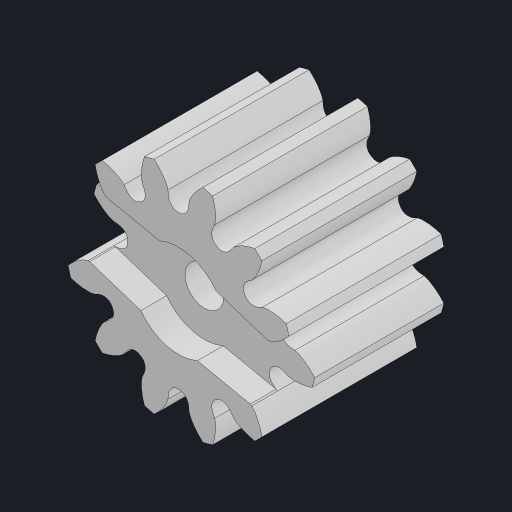
# Autodesk Inventor part: Servo Gear
Saved by Autodesk Inventor 2023.2 (Build 272271030, 271C)
## iProperties
Created: 2023-10-24
Part Number: Servo Gear
Material: Generic
Document SubType Name: Modeling
Designer: robpl
Density: 1 g/cm^3
Appearance: Default
Author: robpl
## iProperties of the stored document Servo Gear_3DPrint.ipt
Created: 2023-10-25
Part Number: Servo Gear_3DPrint
Material: Generic
Document SubType Name: Modeling
Designer: robpl
Density: 1 g/cm^3
Appearance: Default
Author: robpl
Autodesk Inventor part; units mm, degrees
ref_plane "YZ Plane" through (0, 0, 0) normal (1, 0, 0) x (0, 1, 0)
ref_plane "XZ Plane" through (0, 0, 0) normal (0, 1, 0) x (-1, 0, 0)
ref_plane "XY Plane" through (0, 0, 0) normal (0, 0, 1) x (1, 0, 0)
sketch "Sketch1" plane through (0, 0, 0) normal (0, 0, 1) x (1, 0, 0)
  spline S0 degree 3 poles (-1.8876, 8.544) (-1.8289, 8.4914) (-1.7116, 8.3861) (-1.5456, 8.2175) (-1.3882, 8.0411) (-1.2413, 7.8557) (-1.1064, 7.6613) (-1.0062, 7.4915) (-0.9353, 7.3507) (-0.8879, 7.2423) (-0.846, 7.1316) (-0.8276, 7.055) (-0.8183, 7.0166) knots 0 0 0 0 0.125009 0.250019 0.375027 0.500032 0.625031 0.75002 0.812526 0.87503 0.937528 1 1 1 1
  spline S1 degree 3 poles (-0.8183, 7.0166) (-0.8175, 6.9523) (-0.8164, 6.8558) (-0.8022, 6.7278) (-0.7847, 6.6329) (-0.763, 6.5388) (-0.732, 6.4474) (-0.6955, 6.358) (-0.6492, 6.2731) (-0.5944, 6.1935) (-0.5302, 6.1213) (-0.457, 6.058) (-0.3752, 6.0064) (-0.2866, 5.9676) (-0.1929, 5.943) (-0.0964, 5.9357) (0, 5.9384) (0.0964, 5.9357) (0.1929, 5.943) (0.2866, 5.9676) (0.3752, 6.0064) (0.457, 6.058) (0.5302, 6.1213) (0.5944, 6.1935) (0.6492, 6.2731) (0.6955, 6.358) (0.732, 6.4474) (0.763, 6.5388) (0.7847, 6.6329) (0.8022, 6.7278) (0.8164, 6.8558) (0.8175, 6.9523) (0.8183, 7.0166) knots 0 0 0 0 0.062509 0.093773 0.125034 0.156299 0.187559 0.218819 0.250082 0.281336 0.312585 0.343826 0.375061 0.406291 0.43751 0.468735 0.5 0.531265 0.56249 0.593709 0.624939 0.656174 0.687415 0.718664 0.749918 0.781181 0.812441 0.843701 0.874966 0.906227 0.937491 1 1 1 1
  spline S2 degree 3 poles (0.8183, 7.0166) (0.8276, 7.055) (0.846, 7.1316) (0.8879, 7.2423) (0.9353, 7.3507) (1.0062, 7.4915) (1.1064, 7.6613) (1.2413, 7.8557) (1.3882, 8.0411) (1.5456, 8.2175) (1.7116, 8.3861) (1.8289, 8.4914) (1.8876, 8.544) knots 0 0 0 0 0.062472 0.12497 0.187474 0.24998 0.374969 0.499968 0.624973 0.749981 0.874991 1 1 1 1
  circle A0 centre (0, 0) radius 5.9375 construction
  circle A1 centre (0, 0) radius 7.0477 construction
  circle A2 centre (0, 0) radius 7.5 construction
  circle A3 centre (0, 0) radius 8.75
  point P0 (-1.7133, 8.3843)
  point P1 (-1.5471, 8.2162)
  point P2 (-1.3899, 8.0396)
  point P3 (-1.2433, 7.8542)
  point P4 (-1.1089, 7.6597)
  point P5 (-0.9893, 7.4559)
  point P6 (-0.9363, 7.3502)
  point P7 (-0.8889, 7.2419)
  point P8 (-0.8484, 7.1309)
  point P9 (-0.8118, 6.8239)
  point P10 (-0.8011, 6.728)
  point P11 (-0.784, 6.6331)
  point P12 (-0.7615, 6.5393)
  point P13 (-0.7311, 6.4477)
  point P14 (-0.6939, 6.3587)
  point P15 (-0.6478, 6.274)
  point P16 (-0.5928, 6.1948)
  point P17 (-0.5287, 6.1228)
  point P18 (-0.4555, 6.06)
  point P19 (-0.374, 6.0085)
  point P20 (-0.2857, 5.97)
  point P21 (-0.1924, 5.9459)
  point P22 (-0.0965, 5.9373)
  point P23 (0, 5.9375)
  point P24 (0.0965, 5.9373)
  point P25 (0.1924, 5.9459)
  point P26 (0.2857, 5.97)
  point P27 (0.374, 6.0085)
  point P28 (0.4555, 6.06)
  point P29 (0.5287, 6.1228)
  point P30 (0.5928, 6.1948)
  point P31 (0.6478, 6.274)
  point P32 (0.6939, 6.3587)
  point P33 (0.7311, 6.4477)
  point P34 (0.7615, 6.5393)
  point P35 (0.784, 6.6331)
  point P36 (0.8011, 6.728)
  point P37 (0.8118, 6.8239)
  point P38 (0.8484, 7.1309)
  point P39 (0.8889, 7.2419)
  point P40 (0.9363, 7.3502)
  point P41 (0.9893, 7.4559)
  point P42 (1.1089, 7.6597)
  point P43 (1.2433, 7.8542)
  point P44 (1.3899, 8.0396)
  point P45 (1.5471, 8.2162)
  point P46 (1.7133, 8.3843)
  constraints: 4 centre point, 2 point on circle, 109 other
extrude "Extrusion1" add sketch "Sketch1" against normal blind 10
extrude "Extrusion2" cut sketch "Sketch1" against normal through all contours A3 S2 S1 S0 picked at (-0.2347, 7.8651)
pattern_circular "Circular Pattern1" count 12 over 360 about axis through (0, 0, 0) along (0, 0, -1) of "Extrusion2"
sketch "Sketch3" plane through (0, 0, 0) normal (0, 0, 1) x (1, 0, 0)
  spline S0 degree 3 poles (-2.6372, 8.3431) (-2.6618, 8.2682) (-2.7108, 8.1184) (-2.7702, 7.8894) (-2.8183, 7.6579) (-2.8529, 7.4239) (-2.8725, 7.1881) (-2.8743, 6.9909) (-2.8653, 6.8335) (-2.8522, 6.716) (-2.8331, 6.5992) (-2.8108, 6.5235) (-2.7996, 6.4857) knots 0 0 0 0 0.125009 0.250019 0.375027 0.500032 0.625031 0.75002 0.812526 0.87503 0.937528 1 1 1 1 projected
  spline S1 degree 3 poles (-2.7996, 6.4857) (-2.7681, 6.4296) (-2.7209, 6.3455) (-2.6692, 6.2276) (-2.6369, 6.1366) (-2.6086, 6.0443) (-2.5897, 5.9496) (-2.5766, 5.8539) (-2.5743, 5.7573) (-2.582, 5.661) (-2.6015, 5.5663) (-2.6333, 5.4749) (-2.6783, 5.3893) (-2.7356, 5.3114) (-2.8045, 5.2433) (-2.8843, 5.1886) (-2.9692, 5.1428) (-3.0513, 5.0922) (-3.1386, 5.0504) (-3.232, 5.0248) (-3.3281, 5.0141) (-3.4248, 5.0179) (-3.5198, 5.0361) (-3.6115, 5.0666) (-3.6988, 5.1081) (-3.7813, 5.1584) (-3.8576, 5.2176) (-3.9302, 5.2813) (-3.996, 5.3519) (-4.0586, 5.4254) (-4.1349, 5.5291) (-4.1842, 5.6121) (-4.217, 5.6674) knots 0 0 0 0 0.062509 0.093773 0.125034 0.156299 0.187559 0.218819 0.250082 0.281336 0.312585 0.343826 0.375061 0.406291 0.43751 0.468735 0.5 0.531265 0.56249 0.593709 0.624939 0.656174 0.687415 0.718664 0.749918 0.781181 0.812441 0.843701 0.874966 0.906227 0.937491 1 1 1 1 projected
  spline S2 degree 3 poles (-4.217, 5.6674) (-4.2442, 5.696) (-4.2985, 5.7531) (-4.3902, 5.8281) (-4.4853, 5.8982) (-4.6172, 5.9847) (-4.7889, 6.0817) (-5.0028, 6.1826) (-5.2227, 6.2697) (-5.4473, 6.3438) (-5.6753, 6.4068) (-5.8296, 6.4393) (-5.9067, 6.4555) knots 0 0 0 0 0.062472 0.12497 0.187474 0.24998 0.374969 0.499968 0.624973 0.749981 0.874991 1 1 1 1 projected
  arc A0 (-5.9067, 6.4555) -> (-6.4555, 5.9067) centre (0, 0) ccw projected
  spline S3 degree 3 poles (-6.4555, 5.9067) (-6.4393, 5.8296) (-6.4068, 5.6753) (-6.3438, 5.4473) (-6.2697, 5.2227) (-6.1826, 5.0028) (-6.0817, 4.7889) (-5.9847, 4.6172) (-5.8982, 4.4853) (-5.8281, 4.3902) (-5.7531, 4.2985) (-5.696, 4.2442) (-5.6674, 4.217) knots 0 0 0 0 0.125009 0.250019 0.375027 0.500032 0.625031 0.75002 0.812526 0.87503 0.937528 1 1 1 1 projected
  spline S4 degree 3 poles (-5.6674, 4.217) (-5.6121, 4.1842) (-5.5291, 4.1349) (-5.4254, 4.0586) (-5.3519, 3.996) (-5.2813, 3.9302) (-5.2176, 3.8576) (-5.1584, 3.7813) (-5.1081, 3.6988) (-5.0666, 3.6115) (-5.0361, 3.5198) (-5.0179, 3.4248) (-5.0141, 3.3281) (-5.0248, 3.232) (-5.0504, 3.1386) (-5.0922, 3.0513) (-5.1428, 2.9692) (-5.1886, 2.8843) (-5.2433, 2.8045) (-5.3114, 2.7356) (-5.3893, 2.6783) (-5.4749, 2.6333) (-5.5663, 2.6015) (-5.661, 2.582) (-5.7573, 2.5743) (-5.8539, 2.5766) (-5.9496, 2.5897) (-6.0443, 2.6086) (-6.1366, 2.6369) (-6.2276, 2.6692) (-6.3455, 2.7209) (-6.4296, 2.7681) (-6.4857, 2.7996) knots 0 0 0 0 0.062509 0.093773 0.125034 0.156299 0.187559 0.218819 0.250082 0.281336 0.312585 0.343826 0.375061 0.406291 0.43751 0.468735 0.5 0.531265 0.56249 0.593709 0.624939 0.656174 0.687415 0.718664 0.749918 0.781181 0.812441 0.843701 0.874966 0.906227 0.937491 1 1 1 1 projected
  arc A1 (-8.3431, 2.6372) -> (-8.544, 1.8876) centre (0, 0) ccw projected
  spline S5 degree 3 poles (-7.0166, 0.8183) (-6.9523, 0.8175) (-6.8558, 0.8164) (-6.7278, 0.8022) (-6.6329, 0.7847) (-6.5388, 0.763) (-6.4474, 0.732) (-6.358, 0.6955) (-6.2731, 0.6492) (-6.1935, 0.5944) (-6.1213, 0.5302) (-6.058, 0.457) (-6.0064, 0.3752) (-5.9676, 0.2866) (-5.943, 0.1929) (-5.9357, 0.0964) (-5.9384, 0) (-5.9357, -0.0964) (-5.943, -0.1929) (-5.9676, -0.2866) (-6.0064, -0.3752) (-6.058, -0.457) (-6.1213, -0.5302) (-6.1935, -0.5944) (-6.2731, -0.6492) (-6.358, -0.6955) (-6.4474, -0.732) (-6.5388, -0.763) (-6.6329, -0.7847) (-6.7278, -0.8022) (-6.8558, -0.8164) (-6.9523, -0.8175) (-7.0166, -0.8183) knots 0 0 0 0 0.062509 0.093773 0.125034 0.156299 0.187559 0.218819 0.250082 0.281336 0.312585 0.343826 0.375061 0.406291 0.43751 0.468735 0.5 0.531265 0.56249 0.593709 0.624939 0.656174 0.687415 0.718664 0.749918 0.781181 0.812441 0.843701 0.874966 0.906227 0.937491 1 1 1 1 projected
  spline S6 degree 3 poles (-7.0166, -0.8183) (-7.055, -0.8276) (-7.1316, -0.846) (-7.2423, -0.8879) (-7.3507, -0.9353) (-7.4915, -1.0062) (-7.6613, -1.1064) (-7.8557, -1.2413) (-8.0411, -1.3882) (-8.2175, -1.5456) (-8.3861, -1.7116) (-8.4914, -1.8289) (-8.544, -1.8876) knots 0 0 0 0 0.062472 0.12497 0.187474 0.24998 0.374969 0.499968 0.624973 0.749981 0.874991 1 1 1 1 projected
  arc A2 (-8.544, -1.8876) -> (-8.3431, -2.6372) centre (0, 0) ccw projected
  spline S7 degree 3 poles (-8.3431, -2.6372) (-8.2682, -2.6618) (-8.1184, -2.7108) (-7.8894, -2.7702) (-7.6579, -2.8183) (-7.4239, -2.8529) (-7.1881, -2.8725) (-6.9909, -2.8743) (-6.8335, -2.8653) (-6.716, -2.8522) (-6.5992, -2.8331) (-6.5235, -2.8108) (-6.4857, -2.7996) knots 0 0 0 0 0.125009 0.250019 0.375027 0.500032 0.625031 0.75002 0.812526 0.87503 0.937528 1 1 1 1 projected
  spline S8 degree 3 poles (-6.4857, -2.7996) (-6.4296, -2.7681) (-6.3455, -2.7209) (-6.2276, -2.6692) (-6.1366, -2.6369) (-6.0443, -2.6086) (-5.9496, -2.5897) (-5.8539, -2.5766) (-5.7573, -2.5743) (-5.661, -2.582) (-5.5663, -2.6015) (-5.4749, -2.6333) (-5.3893, -2.6783) (-5.3114, -2.7356) (-5.2433, -2.8045) (-5.1886, -2.8843) (-5.1428, -2.9692) (-5.0922, -3.0513) (-5.0504, -3.1386) (-5.0248, -3.232) (-5.0141, -3.3281) (-5.0179, -3.4248) (-5.0361, -3.5198) (-5.0666, -3.6115) (-5.1081, -3.6988) (-5.1584, -3.7813) (-5.2176, -3.8576) (-5.2813, -3.9302) (-5.3519, -3.996) (-5.4254, -4.0586) (-5.5291, -4.1349) (-5.6121, -4.1842) (-5.6674, -4.217) knots 0 0 0 0 0.062509 0.093773 0.125034 0.156299 0.187559 0.218819 0.250082 0.281336 0.312585 0.343826 0.375061 0.406291 0.43751 0.468735 0.5 0.531265 0.56249 0.593709 0.624939 0.656174 0.687415 0.718664 0.749918 0.781181 0.812441 0.843701 0.874966 0.906227 0.937491 1 1 1 1 projected
  spline S9 degree 3 poles (-5.6674, -4.217) (-5.696, -4.2442) (-5.7531, -4.2985) (-5.8281, -4.3902) (-5.8982, -4.4853) (-5.9847, -4.6172) (-6.0817, -4.7889) (-6.1826, -5.0028) (-6.2697, -5.2227) (-6.3438, -5.4473) (-6.4068, -5.6753) (-6.4393, -5.8296) (-6.4555, -5.9067) knots 0 0 0 0 0.062472 0.12497 0.187474 0.24998 0.374969 0.499968 0.624973 0.749981 0.874991 1 1 1 1 projected
  arc A3 (-6.4555, -5.9067) -> (-5.9067, -6.4555) centre (0, 0) ccw projected
  spline S10 degree 3 poles (-5.9067, -6.4555) (-5.8296, -6.4393) (-5.6753, -6.4068) (-5.4473, -6.3438) (-5.2227, -6.2697) (-5.0028, -6.1826) (-4.7889, -6.0817) (-4.6172, -5.9847) (-4.4853, -5.8982) (-4.3902, -5.8281) (-4.2985, -5.7531) (-4.2442, -5.696) (-4.217, -5.6674) knots 0 0 0 0 0.125009 0.250019 0.375027 0.500032 0.625031 0.75002 0.812526 0.87503 0.937528 1 1 1 1 projected
  spline S11 degree 3 poles (-4.217, -5.6674) (-4.1842, -5.6121) (-4.1349, -5.5291) (-4.0586, -5.4254) (-3.996, -5.3519) (-3.9302, -5.2813) (-3.8576, -5.2176) (-3.7813, -5.1584) (-3.6988, -5.1081) (-3.6115, -5.0666) (-3.5198, -5.0361) (-3.4248, -5.0179) (-3.3281, -5.0141) (-3.232, -5.0248) (-3.1386, -5.0504) (-3.0513, -5.0922) (-2.9692, -5.1428) (-2.8843, -5.1886) (-2.8045, -5.2433) (-2.7356, -5.3114) (-2.6783, -5.3893) (-2.6333, -5.4749) (-2.6015, -5.5663) (-2.582, -5.661) (-2.5743, -5.7573) (-2.5766, -5.8539) (-2.5897, -5.9496) (-2.6086, -6.0443) (-2.6369, -6.1366) (-2.6692, -6.2276) (-2.7209, -6.3455) (-2.7681, -6.4296) (-2.7996, -6.4857) knots 0 0 0 0 0.062509 0.093773 0.125034 0.156299 0.187559 0.218819 0.250082 0.281336 0.312585 0.343826 0.375061 0.406291 0.43751 0.468735 0.5 0.531265 0.56249 0.593709 0.624939 0.656174 0.687415 0.718664 0.749918 0.781181 0.812441 0.843701 0.874966 0.906227 0.937491 1 1 1 1 projected
  spline S12 degree 3 poles (-2.7996, -6.4857) (-2.8108, -6.5235) (-2.8331, -6.5992) (-2.8522, -6.716) (-2.8653, -6.8335) (-2.8743, -6.9909) (-2.8725, -7.1881) (-2.8529, -7.4239) (-2.8183, -7.6579) (-2.7702, -7.8894) (-2.7108, -8.1184) (-2.6618, -8.2682) (-2.6372, -8.3431) knots 0 0 0 0 0.062472 0.12497 0.187474 0.24998 0.374969 0.499968 0.624973 0.749981 0.874991 1 1 1 1 projected
  arc A4 (-2.6372, -8.3431) -> (-1.8876, -8.544) centre (0, 0) ccw projected
  spline S13 degree 3 poles (-1.8876, -8.544) (-1.8289, -8.4914) (-1.7116, -8.3861) (-1.5456, -8.2175) (-1.3882, -8.0411) (-1.2413, -7.8557) (-1.1064, -7.6613) (-1.0062, -7.4915) (-0.9353, -7.3507) (-0.8879, -7.2423) (-0.846, -7.1316) (-0.8276, -7.055) (-0.8183, -7.0166) knots 0 0 0 0 0.125009 0.250019 0.375027 0.500032 0.625031 0.75002 0.812526 0.87503 0.937528 1 1 1 1 projected
  spline S14 degree 3 poles (-0.8183, -7.0166) (-0.8175, -6.9523) (-0.8164, -6.8558) (-0.8022, -6.7278) (-0.7847, -6.6329) (-0.763, -6.5388) (-0.732, -6.4474) (-0.6955, -6.358) (-0.6492, -6.2731) (-0.5944, -6.1935) (-0.5302, -6.1213) (-0.457, -6.058) (-0.3752, -6.0064) (-0.2866, -5.9676) (-0.1929, -5.943) (-0.0964, -5.9357) (0, -5.9384) (0.0964, -5.9357) (0.1929, -5.943) (0.2866, -5.9676) (0.3752, -6.0064) (0.457, -6.058) (0.5302, -6.1213) (0.5944, -6.1935) (0.6492, -6.2731) (0.6955, -6.358) (0.732, -6.4474) (0.763, -6.5388) (0.7847, -6.6329) (0.8022, -6.7278) (0.8164, -6.8558) (0.8175, -6.9523) (0.8183, -7.0166) knots 0 0 0 0 0.062509 0.093773 0.125034 0.156299 0.187559 0.218819 0.250082 0.281336 0.312585 0.343826 0.375061 0.406291 0.43751 0.468735 0.5 0.531265 0.56249 0.593709 0.624939 0.656174 0.687415 0.718664 0.749918 0.781181 0.812441 0.843701 0.874966 0.906227 0.937491 1 1 1 1 projected
  spline S15 degree 3 poles (0.8183, -7.0166) (0.8276, -7.055) (0.846, -7.1316) (0.8879, -7.2423) (0.9353, -7.3507) (1.0062, -7.4915) (1.1064, -7.6613) (1.2413, -7.8557) (1.3882, -8.0411) (1.5456, -8.2175) (1.7116, -8.3861) (1.8289, -8.4914) (1.8876, -8.544) knots 0 0 0 0 0.062472 0.12497 0.187474 0.24998 0.374969 0.499968 0.624973 0.749981 0.874991 1 1 1 1 projected
  arc A5 (1.8876, -8.544) -> (2.6372, -8.3431) centre (0, 0) ccw projected
  spline S16 degree 3 poles (2.6372, -8.3431) (2.6618, -8.2682) (2.7108, -8.1184) (2.7702, -7.8894) (2.8183, -7.6579) (2.8529, -7.4239) (2.8725, -7.1881) (2.8743, -6.9909) (2.8653, -6.8335) (2.8522, -6.716) (2.8331, -6.5992) (2.8108, -6.5235) (2.7996, -6.4857) knots 0 0 0 0 0.125009 0.250019 0.375027 0.500032 0.625031 0.75002 0.812526 0.87503 0.937528 1 1 1 1 projected
  spline S17 degree 3 poles (2.7996, -6.4857) (2.7681, -6.4296) (2.7209, -6.3455) (2.6692, -6.2276) (2.6369, -6.1366) (2.6086, -6.0443) (2.5897, -5.9496) (2.5766, -5.8539) (2.5743, -5.7573) (2.582, -5.661) (2.6015, -5.5663) (2.6333, -5.4749) (2.6783, -5.3893) (2.7356, -5.3114) (2.8045, -5.2433) (2.8843, -5.1886) (2.9692, -5.1428) (3.0513, -5.0922) (3.1386, -5.0504) (3.232, -5.0248) (3.3281, -5.0141) (3.4248, -5.0179) (3.5198, -5.0361) (3.6115, -5.0666) (3.6988, -5.1081) (3.7813, -5.1584) (3.8576, -5.2176) (3.9302, -5.2813) (3.996, -5.3519) (4.0586, -5.4254) (4.1349, -5.5291) (4.1842, -5.6121) (4.217, -5.6674) knots 0 0 0 0 0.062509 0.093773 0.125034 0.156299 0.187559 0.218819 0.250082 0.281336 0.312585 0.343826 0.375061 0.406291 0.43751 0.468735 0.5 0.531265 0.56249 0.593709 0.624939 0.656174 0.687415 0.718664 0.749918 0.781181 0.812441 0.843701 0.874966 0.906227 0.937491 1 1 1 1 projected
  spline S18 degree 3 poles (4.217, -5.6674) (4.2442, -5.696) (4.2985, -5.7531) (4.3902, -5.8281) (4.4853, -5.8982) (4.6172, -5.9847) (4.7889, -6.0817) (5.0028, -6.1826) (5.2227, -6.2697) (5.4473, -6.3438) (5.6753, -6.4068) (5.8296, -6.4393) (5.9067, -6.4555) knots 0 0 0 0 0.062472 0.12497 0.187474 0.24998 0.374969 0.499968 0.624973 0.749981 0.874991 1 1 1 1 projected
  arc A6 (5.9067, -6.4555) -> (6.4555, -5.9067) centre (0, 0) ccw projected
  spline S19 degree 3 poles (6.4555, -5.9067) (6.4393, -5.8296) (6.4068, -5.6753) (6.3438, -5.4473) (6.2697, -5.2227) (6.1826, -5.0028) (6.0817, -4.7889) (5.9847, -4.6172) (5.8982, -4.4853) (5.8281, -4.3902) (5.7531, -4.2985) (5.696, -4.2442) (5.6674, -4.217) knots 0 0 0 0 0.125009 0.250019 0.375027 0.500032 0.625031 0.75002 0.812526 0.87503 0.937528 1 1 1 1 projected
  spline S20 degree 3 poles (5.6674, -4.217) (5.6121, -4.1842) (5.5291, -4.1349) (5.4254, -4.0586) (5.3519, -3.996) (5.2813, -3.9302) (5.2176, -3.8576) (5.1584, -3.7813) (5.1081, -3.6988) (5.0666, -3.6115) (5.0361, -3.5198) (5.0179, -3.4248) (5.0141, -3.3281) (5.0248, -3.232) (5.0504, -3.1386) (5.0922, -3.0513) (5.1428, -2.9692) (5.1886, -2.8843) (5.2433, -2.8045) (5.3114, -2.7356) (5.3893, -2.6783) (5.4749, -2.6333) (5.5663, -2.6015) (5.661, -2.582) (5.7573, -2.5743) (5.8539, -2.5766) (5.9496, -2.5897) (6.0443, -2.6086) (6.1366, -2.6369) (6.2276, -2.6692) (6.3455, -2.7209) (6.4296, -2.7681) (6.4857, -2.7996) knots 0 0 0 0 0.062509 0.093773 0.125034 0.156299 0.187559 0.218819 0.250082 0.281336 0.312585 0.343826 0.375061 0.406291 0.43751 0.468735 0.5 0.531265 0.56249 0.593709 0.624939 0.656174 0.687415 0.718664 0.749918 0.781181 0.812441 0.843701 0.874966 0.906227 0.937491 1 1 1 1 projected
  arc A7 (8.3431, -2.6372) -> (8.544, -1.8876) centre (0, 0) ccw projected
  spline S21 degree 3 poles (7.0166, -0.8183) (6.9523, -0.8175) (6.8558, -0.8164) (6.7278, -0.8022) (6.6329, -0.7847) (6.5388, -0.763) (6.4474, -0.732) (6.358, -0.6955) (6.2731, -0.6492) (6.1935, -0.5944) (6.1213, -0.5302) (6.058, -0.457) (6.0064, -0.3752) (5.9676, -0.2866) (5.943, -0.1929) (5.9357, -0.0964) (5.9384, 0) (5.9357, 0.0964) (5.943, 0.1929) (5.9676, 0.2866) (6.0064, 0.3752) (6.058, 0.457) (6.1213, 0.5302) (6.1935, 0.5944) (6.2731, 0.6492) (6.358, 0.6955) (6.4474, 0.732) (6.5388, 0.763) (6.6329, 0.7847) (6.7278, 0.8022) (6.8558, 0.8164) (6.9523, 0.8175) (7.0166, 0.8183) knots 0 0 0 0 0.062509 0.093773 0.125034 0.156299 0.187559 0.218819 0.250082 0.281336 0.312585 0.343826 0.375061 0.406291 0.43751 0.468735 0.5 0.531265 0.56249 0.593709 0.624939 0.656174 0.687415 0.718664 0.749918 0.781181 0.812441 0.843701 0.874966 0.906227 0.937491 1 1 1 1 projected
  spline S22 degree 3 poles (7.0166, 0.8183) (7.055, 0.8276) (7.1316, 0.846) (7.2423, 0.8879) (7.3507, 0.9353) (7.4915, 1.0062) (7.6613, 1.1064) (7.8557, 1.2413) (8.0411, 1.3882) (8.2175, 1.5456) (8.3861, 1.7116) (8.4914, 1.8289) (8.544, 1.8876) knots 0 0 0 0 0.062472 0.12497 0.187474 0.24998 0.374969 0.499968 0.624973 0.749981 0.874991 1 1 1 1 projected
  arc A8 (8.544, 1.8876) -> (8.3431, 2.6372) centre (0, 0) ccw projected
  spline S23 degree 3 poles (8.3431, 2.6372) (8.2682, 2.6618) (8.1184, 2.7108) (7.8894, 2.7702) (7.6579, 2.8183) (7.4239, 2.8529) (7.1881, 2.8725) (6.9909, 2.8743) (6.8335, 2.8653) (6.716, 2.8522) (6.5992, 2.8331) (6.5235, 2.8108) (6.4857, 2.7996) knots 0 0 0 0 0.125009 0.250019 0.375027 0.500032 0.625031 0.75002 0.812526 0.87503 0.937528 1 1 1 1 projected
  spline S24 degree 3 poles (6.4857, 2.7996) (6.4296, 2.7681) (6.3455, 2.7209) (6.2276, 2.6692) (6.1366, 2.6369) (6.0443, 2.6086) (5.9496, 2.5897) (5.8539, 2.5766) (5.7573, 2.5743) (5.661, 2.582) (5.5663, 2.6015) (5.4749, 2.6333) (5.3893, 2.6783) (5.3114, 2.7356) (5.2433, 2.8045) (5.1886, 2.8843) (5.1428, 2.9692) (5.0922, 3.0513) (5.0504, 3.1386) (5.0248, 3.232) (5.0141, 3.3281) (5.0179, 3.4248) (5.0361, 3.5198) (5.0666, 3.6115) (5.1081, 3.6988) (5.1584, 3.7813) (5.2176, 3.8576) (5.2813, 3.9302) (5.3519, 3.996) (5.4254, 4.0586) (5.5291, 4.1349) (5.6121, 4.1842) (5.6674, 4.217) knots 0 0 0 0 0.062509 0.093773 0.125034 0.156299 0.187559 0.218819 0.250082 0.281336 0.312585 0.343826 0.375061 0.406291 0.43751 0.468735 0.5 0.531265 0.56249 0.593709 0.624939 0.656174 0.687415 0.718664 0.749918 0.781181 0.812441 0.843701 0.874966 0.906227 0.937491 1 1 1 1 projected
  spline S25 degree 3 poles (5.6674, 4.217) (5.696, 4.2442) (5.7531, 4.2985) (5.8281, 4.3902) (5.8982, 4.4853) (5.9847, 4.6172) (6.0817, 4.7889) (6.1826, 5.0028) (6.2697, 5.2227) (6.3438, 5.4473) (6.4068, 5.6753) (6.4393, 5.8296) (6.4555, 5.9067) knots 0 0 0 0 0.062472 0.12497 0.187474 0.24998 0.374969 0.499968 0.624973 0.749981 0.874991 1 1 1 1 projected
  arc A9 (6.4555, 5.9067) -> (5.9067, 6.4555) centre (0, 0) ccw projected
  spline S26 degree 3 poles (5.9067, 6.4555) (5.8296, 6.4393) (5.6753, 6.4068) (5.4473, 6.3438) (5.2227, 6.2697) (5.0028, 6.1826) (4.7889, 6.0817) (4.6172, 5.9847) (4.4853, 5.8982) (4.3902, 5.8281) (4.2985, 5.7531) (4.2442, 5.696) (4.217, 5.6674) knots 0 0 0 0 0.125009 0.250019 0.375027 0.500032 0.625031 0.75002 0.812526 0.87503 0.937528 1 1 1 1 projected
  spline S27 degree 3 poles (4.217, 5.6674) (4.1842, 5.6121) (4.1349, 5.5291) (4.0586, 5.4254) (3.996, 5.3519) (3.9302, 5.2813) (3.8576, 5.2176) (3.7813, 5.1584) (3.6988, 5.1081) (3.6115, 5.0666) (3.5198, 5.0361) (3.4248, 5.0179) (3.3281, 5.0141) (3.232, 5.0248) (3.1386, 5.0504) (3.0513, 5.0922) (2.9692, 5.1428) (2.8843, 5.1886) (2.8045, 5.2433) (2.7356, 5.3114) (2.6783, 5.3893) (2.6333, 5.4749) (2.6015, 5.5663) (2.582, 5.661) (2.5743, 5.7573) (2.5766, 5.8539) (2.5897, 5.9496) (2.6086, 6.0443) (2.6369, 6.1366) (2.6692, 6.2276) (2.7209, 6.3455) (2.7681, 6.4296) (2.7996, 6.4857) knots 0 0 0 0 0.062509 0.093773 0.125034 0.156299 0.187559 0.218819 0.250082 0.281336 0.312585 0.343826 0.375061 0.406291 0.43751 0.468735 0.5 0.531265 0.56249 0.593709 0.624939 0.656174 0.687415 0.718664 0.749918 0.781181 0.812441 0.843701 0.874966 0.906227 0.937491 1 1 1 1 projected
  spline S28 degree 3 poles (2.7996, 6.4857) (2.8108, 6.5235) (2.8331, 6.5992) (2.8522, 6.716) (2.8653, 6.8335) (2.8743, 6.9909) (2.8725, 7.1881) (2.8529, 7.4239) (2.8183, 7.6579) (2.7702, 7.8894) (2.7108, 8.1184) (2.6618, 8.2682) (2.6372, 8.3431) knots 0 0 0 0 0.062472 0.12497 0.187474 0.24998 0.374969 0.499968 0.624973 0.749981 0.874991 1 1 1 1 projected
  arc A10 (2.6372, 8.3431) -> (1.8876, 8.544) centre (0, 0) ccw projected
  spline S29 degree 3 poles (1.8876, 8.544) (1.8289, 8.4914) (1.7116, 8.3861) (1.5456, 8.2175) (1.3882, 8.0411) (1.2413, 7.8557) (1.1064, 7.6613) (1.0062, 7.4915) (0.9353, 7.3507) (0.8879, 7.2423) (0.846, 7.1316) (0.8276, 7.055) (0.8183, 7.0166) knots 0 0 0 0 0.125009 0.250019 0.375027 0.500032 0.625031 0.75002 0.812526 0.87503 0.937528 1 1 1 1 projected
  spline S30 degree 3 poles (0.8183, 7.0166) (0.8175, 6.9523) (0.8164, 6.8558) (0.8022, 6.7278) (0.7847, 6.6329) (0.763, 6.5388) (0.732, 6.4474) (0.6955, 6.358) (0.6492, 6.2731) (0.5944, 6.1935) (0.5302, 6.1213) (0.457, 6.058) (0.3752, 6.0064) (0.2866, 5.9676) (0.1929, 5.943) (0.0964, 5.9357) (0, 5.9384) (-0.0964, 5.9357) (-0.1929, 5.943) (-0.2866, 5.9676) (-0.3752, 6.0064) (-0.457, 6.058) (-0.5302, 6.1213) (-0.5944, 6.1935) (-0.6492, 6.2731) (-0.6955, 6.358) (-0.732, 6.4474) (-0.763, 6.5388) (-0.7847, 6.6329) (-0.8022, 6.7278) (-0.8164, 6.8558) (-0.8175, 6.9523) (-0.8183, 7.0166) knots 0 0 0 0 0.062509 0.093773 0.125034 0.156299 0.187559 0.218819 0.250082 0.281336 0.312585 0.343826 0.375061 0.406291 0.43751 0.468735 0.5 0.531265 0.56249 0.593709 0.624939 0.656174 0.687415 0.718664 0.749918 0.781181 0.812441 0.843701 0.874966 0.906227 0.937491 1 1 1 1 projected
  spline S31 degree 3 poles (-0.8183, 7.0166) (-0.8276, 7.055) (-0.846, 7.1316) (-0.8879, 7.2423) (-0.9353, 7.3507) (-1.0062, 7.4915) (-1.1064, 7.6613) (-1.2413, 7.8557) (-1.3882, 8.0411) (-1.5456, 8.2175) (-1.7116, 8.3861) (-1.8289, 8.4914) (-1.8876, 8.544) knots 0 0 0 0 0.062472 0.12497 0.187474 0.24998 0.374969 0.499968 0.624973 0.749981 0.874991 1 1 1 1 projected
  arc A11 (-1.8876, 8.544) -> (-2.6372, 8.3431) centre (0, 0) ccw projected
  circle A12 centre (6.2302, -1.6694) radius 1 projected
  arc A13 (1.4479, -3.1315) -> (2.8197, 1.988) centre (0, 0) ccw projected
  line L0 (13.1598, -5.5936) -> (1.4479, -3.1315) projected
  arc A14 (13.1598, -5.5936) -> (14.1935, -1.7357) centre (13.5713, -3.6364) ccw projected
  line L1 (2.8197, 1.988) -> (14.1935, -1.7357) projected
  circle A15 centre (4.2984, -1.1517) radius 0.6 projected
  circle A16 centre (8.1621, -2.187) radius 0.6 projected
  circle A17 centre (10.0939, -2.7047) radius 0.6 projected
  circle A18 centre (12.0258, -3.2223) radius 0.6 projected
  circle A19 centre (13.9576, -3.7399) radius 0.6 projected
  circle A20 centre (0, 0) radius 3.45 projected
  arc A21 (0.5454, 2.4142) -> (0.4837, 2.4273) centre (0, 0) ccw projected
  line L2 (0.5454, 2.4142) -> (0.6147, 2.2941) projected
  line L3 (0.6147, 2.2941) -> (0.7348, 2.3634) projected
  arc A22 (0.7947, 2.3439) -> (0.7348, 2.3634) centre (0, 0) ccw projected
  line L4 (0.7947, 2.3439) -> (0.8511, 2.2173) projected
  line L5 (0.8511, 2.2173) -> (0.9778, 2.2737) projected
  arc A23 (1.0354, 2.248) -> (0.9778, 2.2737) centre (0, 0) ccw projected
  line L6 (1.0354, 2.248) -> (1.0782, 2.1161) projected
  line L7 (1.0782, 2.1161) -> (1.2101, 2.159) projected
  arc A24 (1.2647, 2.1275) -> (1.2101, 2.159) centre (0, 0) ccw projected
  line L8 (1.2647, 2.1275) -> (1.2935, 1.9918) projected
  line L9 (1.2935, 1.9918) -> (1.4292, 2.0207) projected
  arc A25 (1.4801, 1.9836) -> (1.4292, 2.0207) centre (0, 0) ccw projected
  line L10 (1.4801, 1.9836) -> (1.4946, 1.8457) projected
  line L11 (1.4946, 1.8457) -> (1.6325, 1.8602) projected
  arc A26 (1.6794, 1.8181) -> (1.6325, 1.8602) centre (0, 0) ccw projected
  line L12 (1.6794, 1.8181) -> (1.6794, 1.6794) projected
  line L13 (1.6794, 1.6794) -> (1.8181, 1.6794) projected
  arc A27 (1.8602, 1.6325) -> (1.8181, 1.6794) centre (0, 0) ccw projected
  line L14 (1.8602, 1.6325) -> (1.8457, 1.4946) projected
  line L15 (1.8457, 1.4946) -> (1.9836, 1.4801) projected
  arc A28 (2.0207, 1.4292) -> (1.9836, 1.4801) centre (0, 0) ccw projected
  line L16 (2.0207, 1.4292) -> (1.9918, 1.2935) projected
  line L17 (1.9918, 1.2935) -> (2.1275, 1.2647) projected
  arc A29 (2.159, 1.2101) -> (2.1275, 1.2647) centre (0, 0) ccw projected
  line L18 (2.159, 1.2101) -> (2.1161, 1.0782) projected
  line L19 (2.1161, 1.0782) -> (2.248, 1.0354) projected
  arc A30 (2.2737, 0.9778) -> (2.248, 1.0354) centre (0, 0) ccw projected
  line L20 (2.2737, 0.9778) -> (2.2173, 0.8511) projected
  line L21 (2.2173, 0.8511) -> (2.3439, 0.7947) projected
  arc A31 (2.3634, 0.7348) -> (2.3439, 0.7947) centre (0, 0) ccw projected
  line L22 (2.3634, 0.7348) -> (2.2941, 0.6147) projected
  line L23 (2.2941, 0.6147) -> (2.4142, 0.5454) projected
  arc A32 (2.4273, 0.4837) -> (2.4142, 0.5454) centre (0, 0) ccw projected
  line L24 (2.4273, 0.4837) -> (2.3458, 0.3715) projected
  line L25 (2.3458, 0.3715) -> (2.4579, 0.29) projected
  arc A33 (2.4645, 0.2274) -> (2.4579, 0.29) centre (0, 0) ccw projected
  line L26 (2.4645, 0.2274) -> (2.3717, 0.1243) projected
  line L27 (2.3717, 0.1243) -> (2.4748, 0.0315) projected
  arc A34 (2.4748, -0.0315) -> (2.4748, 0.0315) centre (0, 0) ccw projected
  line L28 (2.4748, -0.0315) -> (2.3717, -0.1243) projected
  line L29 (2.3717, -0.1243) -> (2.4645, -0.2274) projected
  arc A35 (2.4579, -0.29) -> (2.4645, -0.2274) centre (0, 0) ccw projected
  line L30 (2.4579, -0.29) -> (2.3458, -0.3715) projected
  line L31 (2.3458, -0.3715) -> (2.4273, -0.4837) projected
  arc A36 (2.4142, -0.5454) -> (2.4273, -0.4837) centre (0, 0) ccw projected
  line L32 (2.4142, -0.5454) -> (2.2941, -0.6147) projected
  line L33 (2.2941, -0.6147) -> (2.3634, -0.7348) projected
  arc A37 (2.3439, -0.7947) -> (2.3634, -0.7348) centre (0, 0) ccw projected
  line L34 (2.3439, -0.7947) -> (2.2173, -0.8511) projected
  line L35 (2.2173, -0.8511) -> (2.2737, -0.9778) projected
  arc A38 (2.248, -1.0354) -> (2.2737, -0.9778) centre (0, 0) ccw projected
  line L36 (2.248, -1.0354) -> (2.1161, -1.0782) projected
  line L37 (2.1161, -1.0782) -> (2.159, -1.2101) projected
  arc A39 (2.1275, -1.2647) -> (2.159, -1.2101) centre (0, 0) ccw projected
  line L38 (2.1275, -1.2647) -> (1.9918, -1.2935) projected
  line L39 (1.9918, -1.2935) -> (2.0207, -1.4292) projected
  arc A40 (1.9836, -1.4801) -> (2.0207, -1.4292) centre (0, 0) ccw projected
  line L40 (1.9836, -1.4801) -> (1.8457, -1.4946) projected
  line L41 (1.8457, -1.4946) -> (1.8602, -1.6325) projected
  arc A41 (1.8181, -1.6794) -> (1.8602, -1.6325) centre (0, 0) ccw projected
  line L42 (1.8181, -1.6794) -> (1.6794, -1.6794) projected
  line L43 (1.6794, -1.6794) -> (1.6794, -1.8181) projected
  arc A42 (1.6325, -1.8602) -> (1.6794, -1.8181) centre (0, 0) ccw projected
  line L44 (1.6325, -1.8602) -> (1.4946, -1.8457) projected
  line L45 (1.4946, -1.8457) -> (1.4801, -1.9836) projected
  arc A43 (1.4292, -2.0207) -> (1.4801, -1.9836) centre (0, 0) ccw projected
  line L46 (1.4292, -2.0207) -> (1.2935, -1.9918) projected
  line L47 (1.2935, -1.9918) -> (1.2647, -2.1275) projected
  arc A44 (1.2101, -2.159) -> (1.2647, -2.1275) centre (0, 0) ccw projected
  line L48 (1.2101, -2.159) -> (1.0782, -2.1161) projected
  line L49 (1.0782, -2.1161) -> (1.0354, -2.248) projected
  arc A45 (0.9778, -2.2737) -> (1.0354, -2.248) centre (0, 0) ccw projected
  line L50 (0.9778, -2.2737) -> (0.8511, -2.2173) projected
  line L51 (0.8511, -2.2173) -> (0.7947, -2.3439) projected
  arc A46 (0.7348, -2.3634) -> (0.7947, -2.3439) centre (0, 0) ccw projected
  line L52 (0.7348, -2.3634) -> (0.6147, -2.2941) projected
  line L53 (0.6147, -2.2941) -> (0.5454, -2.4142) projected
  arc A47 (0.4837, -2.4273) -> (0.5454, -2.4142) centre (0, 0) ccw projected
  line L54 (0.4837, -2.4273) -> (0.3715, -2.3458) projected
  line L55 (0.3715, -2.3458) -> (0.29, -2.4579) projected
  arc A48 (0.2274, -2.4645) -> (0.29, -2.4579) centre (0, 0) ccw projected
  line L56 (0.2274, -2.4645) -> (0.1243, -2.3717) projected
  line L57 (0.1243, -2.3717) -> (0.0315, -2.4748) projected
  arc A49 (-0.0315, -2.4748) -> (0.0315, -2.4748) centre (0, 0) ccw projected
  line L58 (-0.0315, -2.4748) -> (-0.1243, -2.3717) projected
  line L59 (-0.1243, -2.3717) -> (-0.2274, -2.4645) projected
  arc A50 (-0.29, -2.4579) -> (-0.2274, -2.4645) centre (0, 0) ccw projected
  line L60 (-0.29, -2.4579) -> (-0.3715, -2.3458) projected
  line L61 (-0.3715, -2.3458) -> (-0.4837, -2.4273) projected
  arc A51 (-0.5454, -2.4142) -> (-0.4837, -2.4273) centre (0, 0) ccw projected
  line L62 (-0.5454, -2.4142) -> (-0.6147, -2.2941) projected
  line L63 (-0.6147, -2.2941) -> (-0.7348, -2.3634) projected
  arc A52 (-0.7947, -2.3439) -> (-0.7348, -2.3634) centre (0, 0) ccw projected
  line L64 (-0.7947, -2.3439) -> (-0.8511, -2.2173) projected
  line L65 (-0.8511, -2.2173) -> (-0.9778, -2.2737) projected
  arc A53 (-1.0354, -2.248) -> (-0.9778, -2.2737) centre (0, 0) ccw projected
  line L66 (-1.0354, -2.248) -> (-1.0782, -2.1161) projected
  line L67 (-1.0782, -2.1161) -> (-1.2101, -2.159) projected
  arc A54 (-1.2647, -2.1275) -> (-1.2101, -2.159) centre (0, 0) ccw projected
  line L68 (-1.2647, -2.1275) -> (-1.2935, -1.9918) projected
  line L69 (-1.2935, -1.9918) -> (-1.4292, -2.0207) projected
  arc A55 (-1.4801, -1.9836) -> (-1.4292, -2.0207) centre (0, 0) ccw projected
  line L70 (-1.4801, -1.9836) -> (-1.4946, -1.8457) projected
  line L71 (-1.4946, -1.8457) -> (-1.6325, -1.8602) projected
  arc A56 (-1.6794, -1.8181) -> (-1.6325, -1.8602) centre (0, 0) ccw projected
  line L72 (-1.6794, -1.8181) -> (-1.6794, -1.6794) projected
  line L73 (-1.6794, -1.6794) -> (-1.8181, -1.6794) projected
  arc A57 (-1.8602, -1.6325) -> (-1.8181, -1.6794) centre (0, 0) ccw projected
  line L74 (-1.8602, -1.6325) -> (-1.8457, -1.4946) projected
  line L75 (-1.8457, -1.4946) -> (-1.9836, -1.4801) projected
  arc A58 (-2.0207, -1.4292) -> (-1.9836, -1.4801) centre (0, 0) ccw projected
  line L76 (-2.0207, -1.4292) -> (-1.9918, -1.2935) projected
  line L77 (-1.9918, -1.2935) -> (-2.1275, -1.2647) projected
  arc A59 (-2.159, -1.2101) -> (-2.1275, -1.2647) centre (0, 0) ccw projected
  line L78 (-2.159, -1.2101) -> (-2.1161, -1.0782) projected
  line L79 (-2.1161, -1.0782) -> (-2.248, -1.0354) projected
  arc A60 (-2.2737, -0.9778) -> (-2.248, -1.0354) centre (0, 0) ccw projected
  line L80 (-2.2737, -0.9778) -> (-2.2173, -0.8511) projected
  line L81 (-2.2173, -0.8511) -> (-2.3439, -0.7947) projected
  arc A61 (-2.3634, -0.7348) -> (-2.3439, -0.7947) centre (0, 0) ccw projected
  line L82 (-2.3634, -0.7348) -> (-2.2941, -0.6147) projected
  line L83 (-2.2941, -0.6147) -> (-2.4142, -0.5454) projected
  arc A62 (-2.4273, -0.4837) -> (-2.4142, -0.5454) centre (0, 0) ccw projected
  line L84 (-2.4273, -0.4837) -> (-2.3458, -0.3715) projected
  line L85 (-2.3458, -0.3715) -> (-2.4579, -0.29) projected
  arc A63 (-2.4645, -0.2274) -> (-2.4579, -0.29) centre (0, 0) ccw projected
  line L86 (-2.4645, -0.2274) -> (-2.3717, -0.1243) projected
  line L87 (-2.3717, -0.1243) -> (-2.4748, -0.0315) projected
  arc A64 (-2.4748, 0.0315) -> (-2.4748, -0.0315) centre (0, 0) ccw projected
  line L88 (-2.4748, 0.0315) -> (-2.3717, 0.1243) projected
  line L89 (-2.3717, 0.1243) -> (-2.4645, 0.2274) projected
  arc A65 (-2.4579, 0.29) -> (-2.4645, 0.2274) centre (0, 0) ccw projected
  line L90 (-2.4579, 0.29) -> (-2.3458, 0.3715) projected
  line L91 (-2.3458, 0.3715) -> (-2.4273, 0.4837) projected
  arc A66 (-2.4142, 0.5454) -> (-2.4273, 0.4837) centre (0, 0) ccw projected
  line L92 (-2.4142, 0.5454) -> (-2.2941, 0.6147) projected
  line L93 (-2.2941, 0.6147) -> (-2.3634, 0.7348) projected
  arc A67 (-2.3439, 0.7947) -> (-2.3634, 0.7348) centre (0, 0) ccw projected
  line L94 (-2.3439, 0.7947) -> (-2.2173, 0.8511) projected
  line L95 (-2.2173, 0.8511) -> (-2.2737, 0.9778) projected
  arc A68 (-2.248, 1.0354) -> (-2.2737, 0.9778) centre (0, 0) ccw projected
  line L96 (-2.248, 1.0354) -> (-2.1161, 1.0782) projected
  line L97 (-2.1161, 1.0782) -> (-2.159, 1.2101) projected
  arc A69 (-2.1275, 1.2647) -> (-2.159, 1.2101) centre (0, 0) ccw projected
  line L98 (-2.1275, 1.2647) -> (-1.9918, 1.2935) projected
  line L99 (-1.9918, 1.2935) -> (-2.0207, 1.4292) projected
  arc A70 (-1.9836, 1.4801) -> (-2.0207, 1.4292) centre (0, 0) ccw projected
  line L100 (-1.9836, 1.4801) -> (-1.8457, 1.4946) projected
  line L101 (-1.8457, 1.4946) -> (-1.8602, 1.6325) projected
  arc A71 (-1.8181, 1.6794) -> (-1.8602, 1.6325) centre (0, 0) ccw projected
  line L102 (-1.8181, 1.6794) -> (-1.6794, 1.6794) projected
  line L103 (-1.6794, 1.6794) -> (-1.6794, 1.8181) projected
  arc A72 (-1.6325, 1.8602) -> (-1.6794, 1.8181) centre (0, 0) ccw projected
  line L104 (-1.6325, 1.8602) -> (-1.4946, 1.8457) projected
  line L105 (-1.4946, 1.8457) -> (-1.4801, 1.9836) projected
  arc A73 (-1.4292, 2.0207) -> (-1.4801, 1.9836) centre (0, 0) ccw projected
  line L106 (-1.4292, 2.0207) -> (-1.2935, 1.9918) projected
  line L107 (-1.2935, 1.9918) -> (-1.2647, 2.1275) projected
  arc A74 (-1.2101, 2.159) -> (-1.2647, 2.1275) centre (0, 0) ccw projected
  line L108 (-1.2101, 2.159) -> (-1.0782, 2.1161) projected
  line L109 (-1.0782, 2.1161) -> (-1.0354, 2.248) projected
  arc A75 (-0.9778, 2.2737) -> (-1.0354, 2.248) centre (0, 0) ccw projected
  line L110 (-0.9778, 2.2737) -> (-0.8511, 2.2173) projected
  line L111 (-0.8511, 2.2173) -> (-0.7947, 2.3439) projected
  arc A76 (-0.7348, 2.3634) -> (-0.7947, 2.3439) centre (0, 0) ccw projected
  line L112 (-0.7348, 2.3634) -> (-0.6147, 2.2941) projected
  line L113 (-0.6147, 2.2941) -> (-0.5454, 2.4142) projected
  arc A77 (-0.4837, 2.4273) -> (-0.5454, 2.4142) centre (0, 0) ccw projected
  line L114 (-0.4837, 2.4273) -> (-0.3715, 2.3458) projected
  line L115 (-0.3715, 2.3458) -> (-0.29, 2.4579) projected
  arc A78 (-0.2274, 2.4645) -> (-0.29, 2.4579) centre (0, 0) ccw projected
  line L116 (-0.2274, 2.4645) -> (-0.1243, 2.3717) projected
  line L117 (-0.1243, 2.3717) -> (-0.0315, 2.4748) projected
  arc A79 (0.0315, 2.4748) -> (-0.0315, 2.4748) centre (0, 0) ccw projected
  line L118 (0.0315, 2.4748) -> (0.1243, 2.3717) projected
  line L119 (0.1243, 2.3717) -> (0.2274, 2.4645) projected
  arc A80 (0.29, 2.4579) -> (0.2274, 2.4645) centre (0, 0) ccw projected
  line L120 (0.29, 2.4579) -> (0.3715, 2.3458) projected
  line L121 (0.3715, 2.3458) -> (0.4837, 2.4273) projected
  circle A81 centre (-6.2302, 1.6694) radius 1 projected
  arc A82 (-1.4479, 3.1315) -> (-2.8197, -1.988) centre (0, 0) ccw projected
  line L122 (-13.1598, 5.5936) -> (-1.4479, 3.1315) projected
  arc A83 (-13.1598, 5.5936) -> (-14.1935, 1.7357) centre (-13.5713, 3.6364) ccw projected
  line L123 (-2.8197, -1.988) -> (-14.1935, 1.7357) projected
  circle A84 centre (-10.0939, 2.7047) radius 0.6 projected
  circle A85 centre (-8.1621, 2.187) radius 0.6 projected
  circle A86 centre (-4.2984, 1.1517) radius 0.6 projected
  circle A87 centre (-12.0258, 3.2223) radius 0.6 projected
  circle A88 centre (-13.9576, 3.7399) radius 0.6 projected
  circle A89 centre (0, 0) radius 3.6
  line L124 (1.4652, -3.2884) -> (7.8293, -4.6263)
  line L125 (-2.913, -2.1152) -> (-8.8546, -0.17)
  line L126 (-1.4652, 3.2884) -> (-8.6885, 4.8069)
  line L127 (2.913, 2.1152) -> (8.4014, 0.3184)
  point P0 (5.7966, -4.3522)
  point P1 (-7.1961, -0.8708)
  point P2 (-5.7966, 4.3522)
  point P3 (7.1961, 0.8708)
  point P4 (5.5537, -4.1479)
  point P5 (-6.8836, -0.8153)
  point P6 (6.8836, 0.8153)
  point P7 (-5.5537, 4.1479)
  dimension "d17" = 0.15
  dimension "d18" = 0.15
  dimension "d19" = 0.15
  dimension "d20" = 0.15
  dimension "d21" = 0.15
  constraints: 8 end point, 4 parallel, 4 point on circle, 2 horizontal alignment, 1 centre point, 34 other
  measures "d17" radial gap between concentric circles of A20 A89
  measures "d18" distance between parallel lines of L123 L125
  measures "d19" distance between parallel lines of L122 L126
  measures "d20" distance between parallel lines of L1 L127
  measures "d21" distance between parallel lines of L0 L124
extrude "Extrusion3" add sketch "Sketch3" along normal blind 2 contours A11 S31 S30 S29 A10 S28 S27 S26 A9 S25 S24 S23 A8 S22 S21 L127 A89 L126 S4 S3 A0 S2 S1 S0 | A89 L124 S20 S19 A6 S18 S17 S16 A5 S15 S14 S13 A4 S12 S11 S10 A3 S9 S8 S7 A2 S6 S5 L125
sketch "Sketch4" plane through (0, 0, -10) normal (0, 0, -1) x (-1, 0, 0)
  point P0 (0, 0)
  point P1 (0, 0)
  constraints: 1 coincident
hole "Hole2" at (0, 0, -10) direction (0, 0, 1) diameter 3 end through all counterbore diameter 8 counterbore depth 8
equation "\"d18\" = d17"
equation "\"d19\" = d18"
equation "\"d20\" = d18"
equation "\"d21\" = d18"
equation "\"Module\" = 1.25"
equation "\"PressureAngle\" = 20deg"
equation "\"UnitProfileClearance\" = 0.25"
equation "\"UnitRoundRadius\" = 0.35"
equation "\"HeadDiameter\" = 17.5"
equation "\"RootDiameter\" = 11.875"
equation "\"BaseDiameter\" = 14.09539"
equation "\"PitchDiameter\" = 15"
equation "\"HelixAngle\" = 0"
equation "\"UnitCorrection\" = 0"
equation "\"UnitAddendumModification\" = 0"
equation "\"CircularPitch\" = 3.926991"
equation "\"UnitBacklashShift\" = 0"
equation "\"TotalToolShift\" = 0"
equation "\"IsInternal\" = 0"
body "Solid1"
